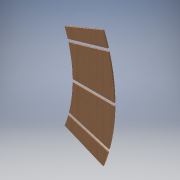
# Autodesk Inventor part: externalSupportRear3
Saved by Autodesk Inventor 2019 (Build 230136000, 136)
## iProperties
Created: 2019-01-12
Part Number: externalSupportRear3
Material: Wood (Cherry)
Document SubType Name: Modeling
Designer: gaincarlo
Density: 0.63 g/cm^3
Appearance: Cherry - Natural Low Gloss
Project: La Panca - Flower Vase
Author: gaincarlo
Autodesk Inventor part; units mm, degrees
ref_plane "YZ Plane" through (0, 0, 0) normal (1, 0, 0) x (0, 1, 0)
ref_plane "XZ Plane" through (0, 0, 0) normal (0, 1, 0) x (-1, 0, 0)
ref_plane "Work Plane1" through (0, 0, 4) normal (0, 0, 1) x (1, 0, 0)
sketch "Sketch1" plane through (0, 0, 4) normal (0, 0, 1) x (1, 0, 0)
  arc A0 (-35.3271, -161.3048) -> (-35.3271, 161.3048) centre (-430, 0) ccw construction
  spline S0 degree 3 poles (-35.3271, 161.3048) (-34.9883, 161.4436) (-34.6494, 161.5824) (-33.9718, 161.86) (-33.633, 161.9988) (-33.2941, 162.1376) knots -0.219692 -0.219692 -0.219692 -0.219692 -0.109846 -0.109846 0 0 0 0 construction
  arc A1 (-33.2941, -162.1376) -> (-33.2941, 162.1376) centre (-430, 0) ccw construction
  spline S1 degree 3 poles (-33.2941, -162.1376) (-33.633, -161.9988) (-33.9718, -161.86) (-34.6494, -161.5824) (-34.9883, -161.4436) (-35.3271, -161.3048) knots -0.219692 -0.219692 -0.219692 -0.219692 -0.109846 -0.109846 0 0 0 0 construction
  line L0 (248.7389, -270.3189) -> (244.912, -279.5577) construction
  line L1 (244.912, -279.5577) -> (-33.5817, -164.2018) construction
  line L2 (-33.5817, -164.2018) -> (-29.7549, -154.963) construction
  line L3 (-29.7549, -154.963) -> (248.7389, -270.3189) construction
  line L4 (275.5471, -193.3679) -> (272.661, -202.9423) construction
  line L5 (272.661, -202.9423) -> (-15.9505, -115.9414) construction
  line L6 (-15.9505, -115.9414) -> (-13.0643, -106.3669) construction
  line L7 (-13.0643, -106.3669) -> (275.5471, -193.3679) construction
  line L8 (300, 5) -> (300, -5) construction
  line L9 (300, -5) -> (-1.4394, -5) construction
  line L10 (-1.4394, -5) -> (-1.4394, 5) construction
  line L11 (-1.4394, 5) -> (300, 5) construction
  line L12 (270.5022, 206.2306) -> (273.3065, 196.6319) construction
  line L13 (273.3065, 196.6319) -> (-16.0379, 112.1006) construction
  line L14 (-16.0379, 112.1006) -> (-18.8422, 121.6993) construction
  line L15 (-18.8422, 121.6993) -> (270.5022, 206.2306) construction
  line L16 (244.5337, 279.401) -> (248.3605, 270.1622) construction
  line L17 (248.3605, 270.1622) -> (-30.1332, 154.8063) construction
  line L18 (-30.1332, 154.8063) -> (-33.9601, 164.0451) construction
  line L19 (-33.9601, 164.0451) -> (244.5337, 279.401) construction
  arc A2 (-30.32, -154.6611) -> (-30.3426, 154.7196) centre (-430, 0) ccw
  arc A3 (108.2672, -212.1337) -> (108.2672, 212.1337) centre (-430, 0) ccw
  line L20 (108.2672, -212.1337) -> (-30.32, -154.6611)
  line L21 (128.9943, -149.19) -> (-14.7215, -105.8674)
  line L22 (148.5389, -5) -> (-1.4686, -5)
  line L23 (148.5389, 5) -> (-1.4686, 5)
  line L24 (127.6654, 154.0832) -> (-16.3369, 112.0132)
  line L25 (124.9189, 163.6988) -> (-19.0631, 121.6348)
  line L26 (108.2672, 212.1337) -> (-30.3426, 154.7196)
  line L27 (126.3315, -158.8318) -> (-17.306, -115.5328)
  point P0 (0, 0)
  dimension "d0" = 150
  constraints: 56 end point, 22 point on circle, 15 point on line, 4 centre point, 2 coincident, 2 horizontal, 2 vertical, 1 collinear, 50 other
  measures "d0" radial gap between concentric circles of A2 A3
extrude "Extrusion1" add sketch "Sketch1" against normal blind 4 contours A2 L27 A3 L20 | A2 L22 A3 L21 | A2 L24 A3 L23 | A2 L26 A3 L25
body "Solid1"
